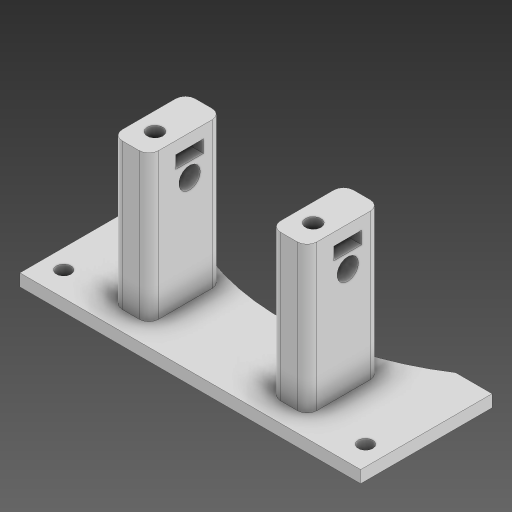
# Autodesk Inventor part: kreplenie_dribler_V2
Saved by Autodesk Inventor 2023 (Build 270158000, 158)
## iProperties
Created: 2025-05-27
Part Number: kreplenie_dribler_V2
Material: Типовые
Document SubType Name: Modeling
Designer: daa
Density: 1 g/cm^3
Appearance: По умолчанию
Author: daa
Autodesk Inventor part; units mm, degrees
ref_plane "YZ Plane" through (0, 0, 0) normal (1, 0, 0) x (0, 1, 0)
ref_plane "XZ Plane" through (0, 0, 0) normal (0, 1, 0) x (-1, 0, 0)
ref_plane "XY Plane" through (0, 0, 0) normal (0, 0, 1) x (1, 0, 0)
sketch "Эскиз1" plane through (0, 0, 0) normal (0, 1, 0) x (-1, 0, 0)
  line L0 (70, -35) -> (62.5, -35)
  line L1 (0, -35) -> (7.5, -35)
  circle A0 centre (66, -13) radius 1.5
  circle A1 centre (4, -13) radius 1.5
  line L2 (70, -8) -> (0, -8)
  line L3 (70, -35) -> (70, -8)
  line L4 (0, -35) -> (0, -8)
  arc A2 (62.5, -35) -> (7.5, -35) centre (35, -76.7582) ccw
  point P0 (0, 0)
  dimension "d4" = 7.5
  dimension "d5" = 7.5
  dimension "d7" = 3
  dimension "d8" = 3
  dimension "d12" = 62
  dimension "d13" = 13
  dimension "d46" = 5
  dimension "d48" = 50
  constraints: 10 end point, 3 centre point, 3 horizontal, 2 point on circle, 1 parallel, 1 vertical
  measures "d4" distance of L0.start L0.end
  measures "d5" distance of L1.start L1.end
  measures "d7" diameter of A0
  measures "d8" diameter of A1
  measures "d12" distance of A1.centre A0.centre
  measures "d13" vertical distance of point (0, 0) A1.centre
  measures "d46" distance from line of L2 A0.centre
  measures "d48" radius of A2
extrude "Выдавливание1" add sketch "Эскиз1" along normal blind 2.5
sketch "Эскиз2" plane through (0, 2.5, 0) normal (0, 1, 0) x (1, 0, 0)
  line L0 (-55, 27) -> (-47.5, 27)
  line L1 (-47.5, 27) -> (-47.5, 12)
  line L2 (-47.5, 12) -> (-55, 12)
  line L3 (-55, 12) -> (-55, 27)
  line L4 (-22.5, 27) -> (-15, 27)
  line L5 (-15, 27) -> (-15, 12)
  line L6 (-15, 12) -> (-22.5, 12)
  line L7 (-22.5, 12) -> (-22.5, 27)
  line L8 (-70, 35) -> (-70, 8) projected
  line L9 (0, 8) -> (0, 35) projected
  point P0 (0, 0)
  point P1 (-60, 0)
  point P2 (-15, 19.5)
  dimension "d17" = 7.5
  dimension "d18" = 15
  dimension "d19" = 7.5
  dimension "d20" = 15
  dimension "d23" = 12
  dimension "d24" = 12
  dimension "d49" = 15
  dimension "d50" = 15
  constraints: 16 end point, 4 parallel, 2 horizontal, 2 perpendicular, 1 midpoint
  measures "d17" distance of L1.end L2.end
  measures "d18" distance of L0.end L1.end
  measures "d19" distance of L5.end L6.end
  measures "d20" distance of L4.end L5.end
  measures "d23" distance from line of L2 point (-60, 0)
  measures "d24" distance from line of point (0, 0) L6
  measures "d49" distance between parallel lines of L3 L8
  measures "d50" distance from line of L9 point (-15, 19.5)
extrude "Выдавливание2" add sketch "Эскиз2" along normal blind 30
sketch "Эскиз3" plane through (-55, 2.5, -27) normal (-1, 0, 0) x (0, 0, 1)
  line L0 (3.8, 27.5) -> (9.5, 27.5)
  line L1 (9.5, 27.5) -> (9.5, 24.9)
  line L2 (9.5, 24.9) -> (3.8, 24.9)
  line L3 (3.8, 24.9) -> (3.8, 27.5)
  line L4 (15, 0) -> (15, 30) projected
  line L5 (0, 30) -> (15, 30) projected
  circle A0 centre (6.65, 22) radius 2.2
  point P0 (27, -2.5)
  dimension "d27" = 5.7
  dimension "d28" = 5.5
  dimension "d29" = 2.6
  dimension "d30" = 2.5
  dimension "d31" = 4.4
  dimension "d32" = 8
  dimension "d51" = 2.85
  constraints: 8 end point, 2 parallel, 1 centre point, 1 horizontal, 1 perpendicular
  measures "d27" distance of L1.end L2.end
  measures "d28" distance between parallel lines of L4 L1
  measures "d29" distance of L0.end L1.end
  measures "d30" distance between parallel lines of L5 L0
  measures "d31" diameter of A0
  measures "d32" distance from line of L5 A0.centre
  measures "d51" horizontal distance of L1.end A0.centre
extrude "Выдавливание3" cut sketch "Эскиз3" against normal blind 41
sketch "Эскиз4" plane through (0, 32.5, 0) normal (0, 1, 0) x (1, 0, 0)
  circle A0 centre (-18.75, 17) radius 1.6
  circle A1 centre (-51.25, 17) radius 1.6
  line L0 (-22.5, 27) -> (-22.5, 12) projected
  line L1 (-22.5, 12) -> (-15, 12) projected
  line L2 (-55, 12) -> (-47.5, 12) projected
  line L3 (-55, 27) -> (-55, 12) projected
  point P0 (0, 0)
  point P1 (-18.75, 12)
  dimension "d35" = 3.2
  dimension "d36" = 3.2
  dimension "d37" = 3.75
  dimension "d38" = 5
  dimension "d39" = 5
  dimension "d40" = 3.75
  constraints: 2 centre point, 1 midpoint
  measures "d35" diameter of A0
  measures "d36" diameter of A1
  measures "d37" distance from line of L0 A0.centre
  measures "d38" distance of point (-18.75, 12) A0.centre
  measures "d39" distance from line of L2 A1.centre
  measures "d40" distance from line of L3 A1.centre
extrude "Выдавливание4" cut sketch "Эскиз4" against normal blind 8
fillet "Сопряжение2" radius 2 8 edges at (-15, 17.5, -27) (-15, 17.5, -12) (-22.5, 17.5, -27) (-22.5, 17.5, -12) (-55, 17.5, -27) (-47.5, 17.5, -27) (-55, 17.5, -12) (-47.5, 17.5, -12)
